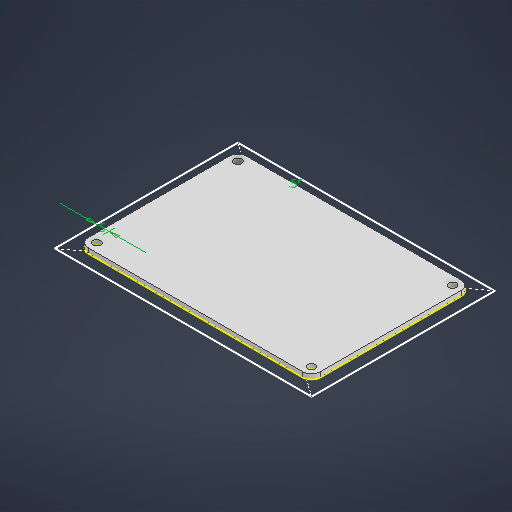
# Autodesk Inventor part: LF_LapTimer-Bottom
Saved by Autodesk Inventor 2026 (Build 300175000, 175)
## iProperties
Created: 2026-03-24
Part Number: LF_LapTimer-Bottom
Material: Všeobecné
Document SubType Name: Modeling
Designer: vadim
Density: 1 g/cm^3
Appearance: Výchozí
Author: vadim
Autodesk Inventor part; units mm, degrees
ref_plane "YZ Plane" through (0, 0, 0) normal (1, 0, 0) x (0, 1, 0)
ref_plane "XZ Plane" through (0, 0, 0) normal (0, 1, 0) x (-1, 0, 0)
ref_plane "XY Plane" through (0, 0, 0) normal (0, 0, 1) x (1, 0, 0)
sketch "Náčrt1" plane through (0, 0, 0) normal (0, 0, 1) x (1, 0, 0)
  line L0 (-43.688, 28.702) -> (43.688, 28.702) construction
  line L1 (43.688, 28.702) -> (43.688, -28.702) construction
  line L2 (43.688, -28.702) -> (-43.688, -28.702) construction
  line L3 (-43.688, -28.702) -> (-43.688, 28.702) construction
  line L4 (-43.688, 28.702) -> (43.688, -28.702) construction
  line L5 (43.688, 28.702) -> (-43.688, -28.702) construction
  circle A0 centre (-43.688, 28.702) radius 1.6
  circle A1 centre (43.688, 28.702) radius 1.6
  circle A2 centre (-43.688, -28.702) radius 1.6
  circle A3 centre (43.688, -28.702) radius 1.6
  line L6 (-43.688, 32.258) -> (43.688, 32.258)
  line L7 (47.244, 28.702) -> (47.244, -28.702)
  line L8 (43.688, -32.258) -> (-43.688, -32.258)
  line L9 (-47.244, -28.702) -> (-47.244, 28.702)
  line L10 (-47.244, 32.258) -> (47.244, -32.258) construction
  line L11 (47.244, 32.258) -> (-47.244, -32.258) construction
  line L12 (0, 28.702) -> (0, -28.702) construction
  line L13 (43.688, 0) -> (-43.688, 0) construction
  arc A4 (-47.244, -28.702) -> (-43.688, -32.258) centre (-43.688, -28.702) ccw
  arc A5 (43.688, -32.258) -> (47.244, -28.702) centre (43.688, -28.702) ccw
  arc A6 (47.244, 28.702) -> (43.688, 32.258) centre (43.688, 28.702) ccw
  arc A7 (-43.688, 32.258) -> (-47.244, 28.702) centre (-43.688, 28.702) ccw
  point P0 (0, 0)
  dimension "d0" = 3.2
  dimension "d1" = 87.376
  dimension "d2" = 94.488
  dimension "d3" = 64.516
  dimension "d5" = 57.404
  dimension "d6" = 3.2
  dimension "d7" = 3.556
  constraints: 28 end point, 8 centre point, 8 midpoint, 8 point on circle, 8 point on line, 8 tangent, 4 coincident, 4 parallel, 3 equal radius, 2 horizontal, 2 perpendicular, 2 other
  measures "d0" diameter of A0
  measures "d1" distance of L0.start L0.end
  measures "d2" distance between parallel lines of L7 L9
  measures "d3" distance between parallel lines of L6 L8
  measures "d5" distance between parallel lines of L2 L0
  measures "d6" diameter of A2
  measures "d7" radius of A4
extrude "Vysunutí1" add sketch "Náčrt1" along normal blind 2
sketch "Náčrt2" plane through (0, 0, 0) normal (0, 0, -1) x (-1, 0, 0)
  circle A0 centre (43.688, -28.702) radius 1.6 projected
  line L0 (43.688, -32.258) -> (-43.688, -32.258) projected
  arc A1 (43.688, -32.258) -> (47.244, -28.702) centre (43.688, -28.702) ccw projected
  line L1 (47.244, 28.702) -> (47.244, -28.702) projected
  arc A2 (47.244, 28.702) -> (43.688, 32.258) centre (43.688, 28.702) ccw projected
  line L2 (-43.688, 32.258) -> (43.688, 32.258) projected
  arc A3 (-43.688, 32.258) -> (-47.244, 28.702) centre (-43.688, 28.702) ccw projected
  line L3 (-47.244, -28.702) -> (-47.244, 28.702) projected
  arc A4 (-47.244, -28.702) -> (-43.688, -32.258) centre (-43.688, -28.702) ccw projected
  circle A5 centre (-43.688, -28.702) radius 1.6 projected
  circle A6 centre (43.688, -28.702) radius 1.6 projected
  circle A7 centre (-43.688, 28.702) radius 1.6 projected
  circle A8 centre (43.688, 28.702) radius 1.6 projected
  line L4 (52.244, -37.258) -> (-52.244, -37.258)
  line L5 (-52.244, -37.258) -> (-52.244, 37.258)
  line L6 (-52.244, 37.258) -> (52.244, 37.258)
  line L7 (52.244, 37.258) -> (52.244, -37.258)
  line L8 (52.244, -37.258) -> (-52.244, 37.258) construction
  line L9 (-52.244, -37.258) -> (52.244, 37.258) construction
  point P0 (0, 0)
  dimension "d10" = 5
  dimension "d11" = 5
  constraints: 12 end point, 2 midpoint, 2 parallel, 1 horizontal, 1 perpendicular
  measures "d10" distance between parallel lines of L7 L1
  measures "d11" distance between parallel lines of L2 L6
